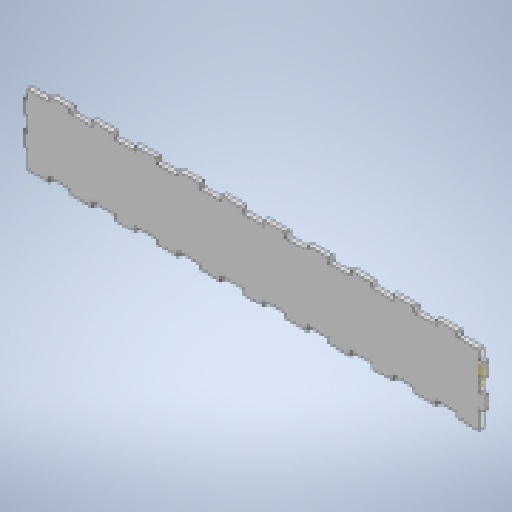
# Autodesk Inventor part: BackWall
Saved by Autodesk Inventor 2024 (Build 280153000, 153)
## iProperties
Created: 2023-09-10
Part Number: BackWall
Material: Generic
Document SubType Name: Modeling
Designer: Bruno
Density: 1 g/cm^3
Appearance: Default
Author: Bruno
Autodesk Inventor part; units mm, degrees
ref_plane "YZ Plane" through (0, 0, 0) normal (1, 0, 0) x (0, 1, 0)
ref_plane "XZ Plane" through (0, 0, 0) normal (0, 1, 0) x (-1, 0, 0)
ref_plane "XY Plane" through (0, 0, 0) normal (0, 0, 1) x (1, 0, 0)
ref_plane "Work Plane1" through (139.4467, 111.518, -98.9659) normal (0, 0, -1) x (-1, 0, 0)
sketch "Sketch1" plane through (139.4467, 111.518, -98.9659) normal (0, 0, -1) x (-1, 0, 0)
  line L0 (0, -27.375) -> (14, -27.375)
  line L1 (14, -27.375) -> (14, -24.375)
  line L2 (14, -24.375) -> (28, -24.375)
  line L3 (28, -24.375) -> (28, -27.375)
  line L4 (56, -24.375) -> (56, -27.375)
  line L5 (42, -24.375) -> (56, -24.375)
  line L6 (42, -27.375) -> (42, -24.375)
  line L7 (28, -27.375) -> (42, -27.375)
  line L8 (84, -24.375) -> (84, -27.375)
  line L9 (70, -24.375) -> (84, -24.375)
  line L10 (70, -27.375) -> (70, -24.375)
  line L11 (56, -27.375) -> (70, -27.375)
  line L12 (112, -24.375) -> (112, -27.375)
  line L13 (98, -24.375) -> (112, -24.375)
  line L14 (98, -27.375) -> (98, -24.375)
  line L15 (84, -27.375) -> (98, -27.375)
  line L16 (140, -24.375) -> (140, -27.375)
  line L17 (126, -24.375) -> (140, -24.375)
  line L18 (126, -27.375) -> (126, -24.375)
  line L19 (112, -27.375) -> (126, -27.375)
  line L20 (168, -24.375) -> (168, -27.375)
  line L21 (154, -24.375) -> (168, -24.375)
  line L22 (154, -27.375) -> (154, -24.375)
  line L23 (140, -27.375) -> (154, -27.375)
  line L24 (196, -24.375) -> (196, -27.375)
  line L25 (182, -24.375) -> (196, -24.375)
  line L26 (182, -27.375) -> (182, -24.375)
  line L27 (168, -27.375) -> (182, -27.375)
  line L28 (224, -24.375) -> (224, -27.375)
  line L29 (210, -24.375) -> (224, -24.375)
  line L30 (210, -27.375) -> (210, -24.375)
  line L31 (196, -27.375) -> (210, -27.375)
  line L32 (252, -24.375) -> (252, -27.375)
  line L33 (238, -24.375) -> (252, -24.375)
  line L34 (238, -27.375) -> (238, -24.375)
  line L35 (224, -27.375) -> (238, -27.375)
  line L36 (280, -24.375) -> (280, -27.375)
  line L37 (266, -24.375) -> (280, -24.375)
  line L38 (266, -27.375) -> (266, -24.375)
  line L39 (252, -27.375) -> (266, -27.375)
  line L40 (280, -27.375) -> (294, -27.375)
  line L41 (0, 18.25) -> (14, 18.25)
  line L42 (14, 18.25) -> (14, 21.25)
  line L43 (14, 21.25) -> (28, 21.25)
  line L44 (28, 21.25) -> (28, 18.25)
  line L45 (56, 21.25) -> (56, 18.25)
  line L46 (42, 21.25) -> (56, 21.25)
  line L47 (42, 18.25) -> (42, 21.25)
  line L48 (28, 18.25) -> (42, 18.25)
  line L49 (84, 21.25) -> (84, 18.25)
  line L50 (70, 21.25) -> (84, 21.25)
  line L51 (70, 18.25) -> (70, 21.25)
  line L52 (56, 18.25) -> (70, 18.25)
  line L53 (112, 21.25) -> (112, 18.25)
  line L54 (98, 21.25) -> (112, 21.25)
  line L55 (98, 18.25) -> (98, 21.25)
  line L56 (84, 18.25) -> (98, 18.25)
  line L57 (140, 21.25) -> (140, 18.25)
  line L58 (126, 21.25) -> (140, 21.25)
  line L59 (126, 18.25) -> (126, 21.25)
  line L60 (112, 18.25) -> (126, 18.25)
  line L61 (168, 21.25) -> (168, 18.25)
  line L62 (154, 21.25) -> (168, 21.25)
  line L63 (154, 18.25) -> (154, 21.25)
  line L64 (140, 18.25) -> (154, 18.25)
  line L65 (196, 21.25) -> (196, 18.25)
  line L66 (182, 21.25) -> (196, 21.25)
  line L67 (182, 18.25) -> (182, 21.25)
  line L68 (168, 18.25) -> (182, 18.25)
  line L69 (224, 21.25) -> (224, 18.25)
  line L70 (210, 21.25) -> (224, 21.25)
  line L71 (210, 18.25) -> (210, 21.25)
  line L72 (196, 18.25) -> (210, 18.25)
  line L73 (252, 21.25) -> (252, 18.25)
  line L74 (238, 21.25) -> (252, 21.25)
  line L75 (238, 18.25) -> (238, 21.25)
  line L76 (224, 18.25) -> (238, 18.25)
  line L77 (280, 21.25) -> (280, 18.25)
  line L78 (266, 21.25) -> (280, 21.25)
  line L79 (266, 18.25) -> (266, 21.25)
  line L80 (252, 18.25) -> (266, 18.25)
  line L81 (280, 18.25) -> (294, 18.25)
  line L82 (297, 12.125) -> (297, 3)
  line L83 (297, 3) -> (294, 3)
  line L84 (294, 3) -> (294, -6.125)
  line L85 (297, -6.125) -> (294, -6.125)
  line L86 (297, -6.125) -> (297, -15.25)
  line L87 (297, -15.25) -> (294, -15.25)
  line L88 (294, -15.25) -> (294, -24.375)
  line L89 (297, 12.125) -> (294, 12.125)
  line L90 (0, -15.25) -> (0, -24.375)
  line L91 (0, -15.25) -> (-3, -15.25)
  line L92 (-3, -6.125) -> (-3, -15.25)
  line L93 (0, -6.125) -> (-3, -6.125)
  line L94 (0, 3) -> (0, -6.125)
  line L95 (0, 3) -> (-3, 3)
  line L96 (-3, 12.125) -> (-3, 3)
  line L97 (0, 12.125) -> (-3, 12.125)
  line L98 (0, -27.375) -> (0, -24.375)
  line L99 (0, 12.125) -> (0, 18.25)
  line L100 (294, -27.375) -> (294, -24.375)
  line L101 (294, 12.125) -> (294, 18.25)
  line L102 (294, 21.25) -> (-3, 21.25)
  point P0 (139.4467, -111.518)
  point P1 (28, -27.375)
  point P2 (56, -27.375)
  point P3 (168, -27.375)
  point P4 (224, -27.375)
  point P5 (252, 18.25)
  point P6 (224, 18.25)
  point P7 (196, 18.25)
  point P8 (168, 18.25)
  point P9 (140, 18.25)
  point P10 (112, 18.25)
  point P11 (84, 18.25)
  point P12 (56, 18.25)
  point P13 (28, 18.25)
  dimension "d0" = 3
  dimension "d1" = 14
  dimension "d4" = 28
  dimension "d13" = 3
  dimension "d14" = 14
  dimension "d15" = 28
  constraints: 204 end point, 20 point on line, 14 horizontal, 10 vertical, 7 perpendicular, 3 collinear, 2 parallel, 184 other
  measures "d0" distance of L0.end L1.end
  measures "d1" distance of L0.start L0.end
  measures "d4" distance of L2.end L4.start
  measures "d13" distance of L42.start L43.start
  measures "d14" distance of L41.start L42.start
  measures "d15" distance of L44.start L46.end
extrude "Extrusion1" add sketch "Sketch1" along normal blind 3 contours L98 L90 L91 L92 L93 L94 L95 L96 L97 L99 L41 L42 L43 L44 L48 L47 L46 L45 L52 L51 L50 L49 L56 L55 L54 L53 L60 L59 L58 L57 L64 L63 L62 L61 L68 L67 L66 L65 L72 L71 L70 L69 L76 L75 L74 L73 L80 L79 L78 L77 L81 L101 L89 L82 L83 L84 L85 L86 L87 L88 L100 L40 L36 L37 L38 L39 L32 L33 L34 L35 L28 L29 L30 L31 L24 L25 L26 L27 L20 L21 L22 L23 L16 L17 L18 L19 L12 L13 L14 L15 L8 L9 L10 L11 L4 L5 L6 L7 L3 L2 L1 L0
body "Solid1"
